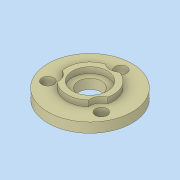
# Autodesk Inventor part: bearingHousing
Saved by Autodesk Inventor 2017 (Build 210142000, 142)
## iProperties
Created: 2016-10-29
Part Number: bearingHousing
Material: ABS Plastic
Document SubType Name: Modeling
Designer: techn
Density: 1.06 g/cm^3
Appearance: Smooth - Ash
Author: techn
Autodesk Inventor part; units mm, degrees
ref_plane "YZ Plane" through (0, 0, 0) normal (1, 0, 0) x (0, 1, 0)
ref_plane "XZ Plane" through (0, 0, 0) normal (0, 1, 0) x (-1, 0, 0)
ref_plane "XY Plane" through (0, 0, 0) normal (0, 0, 1) x (1, 0, 0)
sketch "Sketch7" plane through (0, 0, 0) normal (0, 1, 0) x (-1, 0, 0)
  line L0 (0, 0) -> (0, -7.9375)
  circle A0 centre (0, -7.9375) radius 1.524
  circle A1 centre (0, 0) radius 3
  circle A2 centre (6.8741, 3.9687) radius 1.524
  circle A3 centre (-6.8741, 3.9688) radius 1.524
  circle A4 centre (0, 0) radius 10.795
  dimension "d32" = 7.9375
  dimension "d33" = 3.048
  dimension "d34" = 6
  dimension "d37" = 360
  dimension "d39" = 21.59
  constraints: 5 centre point, 3 coincident, 2 end point, 1 vertical, 7 other
  measures "d32" distance of L0.start L0.end
  measures "d33" diameter of A0
  measures "d34" diameter of A1
  measures "d39" diameter of A4
extrude "Extrusion6" add sketch "Sketch7" along normal blind 2.5
sketch "Sketch8" plane through (0, 2.5, 0) normal (0, 1, 0) x (1, 0, 0)
  circle A0 centre (0, 0) radius 4.5
  circle A1 centre (0, 0) radius 6
  dimension "d42" = 9
  dimension "d43" = 12
  constraints: 2 centre point, 2 coincident
  measures "d42" diameter of A0
  measures "d43" diameter of A1
extrude "Extrusion7" add sketch "Sketch8" along normal blind 1.5
sketch "Sketch9" plane through (0, 2.5, 0) normal (0, 1, 0) x (1, 0, 0)
  circle A0 centre (0, 7.9375) radius 1.524 projected
  circle A1 centre (0, 7.9375) radius 2.8575
  circle A2 centre (-6.8741, -3.9687) radius 2.8575
  circle A3 centre (6.8741, -3.9688) radius 2.8575
  point P0 (0, 0)
  dimension "d46" = 5.715
  dimension "d49" = 360
  constraints: 3 centre point, 1 coincident, 7 other
  measures "d46" diameter of A1
extrude "Extrusion8" cut sketch "Sketch9" along normal blind 1.5
body "Solid2"
